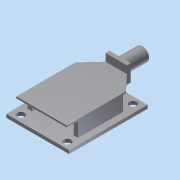
# Autodesk Inventor part: XBee
Saved by Autodesk Inventor 2011 SP1 (Build 150282100, 282)
## iProperties
Created: 2011-08-14
Part Number: XBee
Document SubType Name: Modeling
Designer: dgitz
Density: 1 g/cm^3
Author: dgitz
Autodesk Inventor part; units mm, degrees
ref_plane "YZ Plane" through (0, 0, 0) normal (1, 0, 0) x (0, 1, 0)
ref_plane "XZ Plane" through (0, 0, 0) normal (0, 1, 0) x (-1, 0, 0)
ref_plane "XY Plane" through (0, 0, 0) normal (0, 0, 1) x (1, 0, 0)
sketch "Sketch2" plane through (0, 0, 0) normal (0, 1, 0) x (-1, 0, 0)
  line L0 (-14.224, 17.78) -> (14.224, 17.78)
  line L1 (14.224, 17.78) -> (14.224, -17.78)
  line L2 (14.224, -17.78) -> (-14.224, -17.78)
  line L3 (-14.224, -17.78) -> (-14.224, 17.78)
  circle A0 centre (-10.541, 14.859) radius 1.651
  circle A1 centre (-10.541, -14.859) radius 1.651
  line L4 (0, 13.208) -> (0, -8.1739) construction
  circle A2 centre (10.541, 14.859) radius 1.651
  circle A3 centre (10.541, -14.859) radius 1.651
  point P0 (0, 0)
  dimension "d0" = 28.448
  dimension "d1" = 35.56
  dimension "d2" = 14.224
  dimension "d3" = 17.78
  dimension "d4" = 3.302
  dimension "d5" = 1.27
  dimension "d6" = 2.032
  dimension "d7" = 3.302
  dimension "d8" = 1.27
  dimension "d9" = 2.032
  constraints: 10 end point, 4 centre point, 3 parallel, 2 symmetric about line, 1 horizontal, 1 perpendicular, 2 other
  measures "d0" distance of L1.end L2.end
  measures "d1" distance between parallel lines of L2 L0
  measures "d2" distance from line of point (0, 0) L3
  measures "d3" distance from line of point (0, 0) L0
  measures "d4" diameter of A0
  measures "d5" distance edge to line of A0 L0
  measures "d6" distance edge to line of A0 L3
  measures "d7" diameter of A1
  measures "d8" distance edge to line of A1 L2
  measures "d9" distance edge to line of A1 L3
extrude "Extrusion1" add sketch "Sketch2" along normal blind 1.524
sketch "Sketch3" plane through (0, 1.524, 0) normal (0, 1, 0) x (1, 0, 0)
  line L0 (-14.224, -17.78) -> (-14.224, 17.78) projected
  line L1 (-14.224, 17.78) -> (14.224, 17.78) projected
  line L2 (-11.43, 9.398) -> (-9.398, 9.398)
  line L3 (-9.398, 9.398) -> (-9.398, -10.922)
  line L4 (-9.398, -10.922) -> (-11.43, -10.922)
  line L5 (-11.43, -10.922) -> (-11.43, 9.398)
  line L6 (0, 9.398) -> (0, -9.2858) construction
  line L7 (11.43, 9.398) -> (9.398, 9.398)
  line L8 (9.398, 9.398) -> (9.398, -10.922)
  line L9 (9.398, -10.922) -> (11.43, -10.922)
  line L10 (11.43, -10.922) -> (11.43, 9.398)
  point P0 (0, 0)
  dimension "d12" = 2.032
  dimension "d13" = 20.32
  dimension "d14" = 2.794
  dimension "d15" = 8.382
  constraints: 18 end point, 4 symmetric about line, 3 parallel, 1 horizontal, 1 perpendicular
  measures "d12" distance between parallel lines of L3 L5
  measures "d13" distance between parallel lines of L4 L2
  measures "d14" distance between parallel lines of L0 L5
  measures "d15" distance between parallel lines of L2 L1
extrude "Extrusion2" add sketch "Sketch3" along normal blind 6.604
sketch "Sketch4" plane through (0, 8.128, 0) normal (0, 1, 0) x (1, 0, 0)
  line L0 (-9.398, 9.398) -> (-9.398, -10.922) projected
  line L1 (-11.43, 9.398) -> (-9.398, 9.398) projected
  line L2 (-11.43, -10.922) -> (-11.43, 9.398) projected
  line L3 (-9.398, -10.922) -> (-11.43, -10.922) projected
  line L4 (11.43, 10.668) -> (11.43, -16.002)
  line L5 (11.43, -16.002) -> (-11.43, -16.002)
  line L6 (-11.43, -16.002) -> (-11.43, 10.668)
  line L7 (-11.43, 10.668) -> (-4.826, 17.78)
  line L8 (-4.826, 17.78) -> (4.826, 17.78)
  line L9 (-14.224, -17.78) -> (-14.224, 17.78) projected
  line L10 (4.826, 17.78) -> (11.43, 10.668)
  line L11 (-11.43, 5.9569) -> (-11.43, -5.9458) construction
  line L12 (14.224, 17.78) -> (14.224, -17.78) construction
  point P0 (0, 0)
  dimension "d18" = 2.794
  dimension "d19" = 2.794
  dimension "d20" = 5.08
  dimension "d21" = 9.652
  dimension "d23" = 26.67
  dimension "d24" = 42.879
  dimension "d25" = 137.121
  dimension "d26" = 16.8789
  dimension "d27" = 4.9762
  constraints: 14 end point, 2 point on line, 1 equal length, 1 parallel, 1 perpendicular
  measures "d18" distance between parallel lines of L6 L9
  measures "d19" distance between parallel lines of L12 L4
  measures "d20" distance between parallel lines of L5 L3
  measures "d21" distance of L8.end L7.end
  measures "d23" distance from line of L5 L6.end
  measures "d24" angle of L0 L10
  measures "d25" angle of L0 L7
  measures "d26" distance from line of L11.start L3
  measures "d27" distance from line of L11.end L3
extrude "Extrusion3" add sketch "Sketch4" along normal blind 0.762
sketch "Sketch5" plane through (4.826, 8.128, -17.78) normal (0, 0, -1) x (-1, 0, 0)
  line L0 (9.652, 0.762) -> (0, 0.762) projected
  line L1 (0, 0) -> (0, 0.762) projected
  line L2 (9.652, 0) -> (9.652, 0.762) projected
  line L3 (0, 4.191) -> (9.652, 4.191)
  line L4 (9.652, 4.191) -> (9.652, -3.429)
  line L5 (9.652, -3.429) -> (0, -3.429)
  line L6 (0, -3.429) -> (0, 4.191)
  point P0 (4.826, -8.128)
  point P1 (0, 0.381)
  point P2 (9.652, 0.381)
  dimension "d30" = 7.62
  dimension "d31" = 3.429
  constraints: 8 end point, 4 midpoint, 2 parallel, 1 horizontal, 1 perpendicular
  measures "d30" distance between parallel lines of L5 L3
  measures "d31" distance between parallel lines of L0 L3
extrude "Extrusion4" add sketch "Sketch5" along normal blind 1.778
sketch "Sketch6" plane through (4.826, 8.128, -19.558) normal (0, 0, -1) x (-1, 0, 0)
  circle A0 centre (4.826, 0.381) radius 3.048
  line L0 (0, 4.191) -> (9.652, -3.429) construction
  point P0 (4.826, -8.128)
  point P1 (4.826, 0.381)
  dimension "d34" = 6.096
  constraints: 2 end point, 1 centre point, 1 coincident, 1 midpoint
  measures "d34" diameter of A0
extrude "Extrusion5" add sketch "Sketch6" along normal blind 10.033
body "Solid1"
